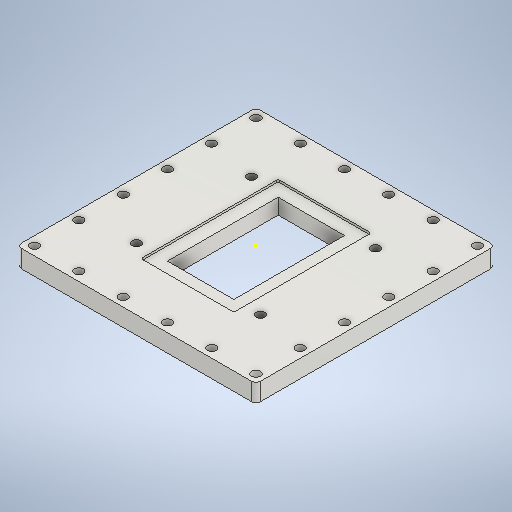
# Autodesk Inventor part: Impact Test Fixturev4 BS EN 6038 assemblyFEA
Saved by Autodesk Inventor 2025 (Build 290162000, 162)
## iProperties
Created: 2024-10-03
Part Number: Impact Test Fixturev4 BS EN 6038 assemblyFEA
Material: Steel, Carbon
Document SubType Name: Modeling
Designer: dr1e22
Density: 7.85 g/cm^3
Appearance: Steel
Author: dr1e22
Autodesk Inventor part; units mm, degrees
ref_plane "YZ Plane" through (0, 0, 0) normal (1, 0, 0) x (0, 1, 0)
ref_plane "XZ Plane" through (0, 0, 0) normal (0, 1, 0) x (-1, 0, 0)
ref_plane "XY Plane" through (0, 0, 0) normal (0, 0, 1) x (1, 0, 0)
sketch "Sketch1" plane through (0, 0, 0) normal (0, 1, 0) x (-1, 0, 0)
  line L0 (130, 135) -> (-130, 135)
  line L1 (-135, 130) -> (-135, -130)
  line L2 (-130, -135) -> (130, -135)
  line L3 (135, -130) -> (135, 130)
  line L4 (135, 135) -> (-135, -135) construction
  line L5 (-135, 135) -> (135, -135) construction
  arc A0 (135, 130) -> (130, 135) centre (130, 130) ccw
  arc A1 (130, -135) -> (135, -130) centre (130, -130) ccw
  arc A2 (-135, -130) -> (-130, -135) centre (-130, -130) ccw
  arc A3 (-130, 135) -> (-135, 130) centre (-130, 130) ccw
  point P0 (0, 0)
  point P1 (0, 0)
  dimension "d0" = 270
  dimension "d1" = 270
  dimension "d2" = 5
  dimension "d3" = 5
  dimension "d4" = 5
  dimension "d5" = 5
  constraints: 12 end point, 8 point on circle, 8 point on line, 8 tangent, 4 centre point, 2 midpoint, 2 parallel, 1 coincident, 1 horizontal, 1 perpendicular
  measures "d0" distance of L4.end L5.end
  measures "d1" distance of L5.end L4.start
  measures "d2" radius of A0
  measures "d3" radius of A1
  measures "d4" radius of A2
  measures "d5" radius of A3
extrude "Extrusion1" add sketch "Sketch1" along normal blind 20
sketch "Sketch2" plane through (0, 20, 0) normal (0, 1, 0) x (1, 0, 0)
  line L0 (-37.5, -62.5) -> (37.5, -62.5)
  line L1 (37.5, -62.5) -> (37.5, 62.5)
  line L2 (37.5, 62.5) -> (-37.5, 62.5)
  line L3 (-37.5, 62.5) -> (-37.5, -62.5)
  line L4 (-37.5, -62.5) -> (37.5, 62.5) construction
  line L5 (37.5, -62.5) -> (-37.5, 62.5) construction
  point P0 (0, 0)
  dimension "d8" = 75
  dimension "d9" = 125
  constraints: 12 end point, 2 midpoint, 2 parallel, 1 horizontal, 1 perpendicular
  measures "d8" distance of L1.end L2.end
  measures "d9" distance of L0.end L1.end
extrude "Extrusion2" cut sketch "Sketch2" against normal blind 65.25
sketch "Sketch3" plane through (0, 20, 0) normal (0, 1, 0) x (1, 0, 0)
  line L0 (-50.5, -77.5) -> (50.5, -77.5)
  line L1 (52.5, -75.5) -> (52.5, 75.5)
  line L2 (50.5, 77.5) -> (-50.5, 77.5)
  line L3 (-52.5, 75.5) -> (-52.5, -75.5)
  line L4 (-52.5, -77.5) -> (52.5, 77.5) construction
  line L5 (52.5, -77.5) -> (-52.5, 77.5) construction
  arc A0 (-50.5, 77.5) -> (-52.5, 75.5) centre (-50.5, 75.5) ccw
  arc A1 (52.5, 75.5) -> (50.5, 77.5) centre (50.5, 75.5) ccw
  arc A2 (50.5, -77.5) -> (52.5, -75.5) centre (50.5, -75.5) ccw
  arc A3 (-52.5, -75.5) -> (-50.5, -77.5) centre (-50.5, -75.5) ccw
  point P0 (0, 0)
  dimension "d12" = 105
  dimension "d13" = 155
  dimension "d14" = 2
  constraints: 12 end point, 8 point on circle, 8 point on line, 8 tangent, 4 centre point, 3 equal radius, 2 midpoint, 2 parallel, 1 horizontal, 1 perpendicular
  measures "d12" distance of L4.end L5.end
  measures "d13" distance of L5.start L4.end
  measures "d14" radius of A0
extrude "Extrusion3" cut sketch "Sketch3" against normal blind 2.5
sketch "Sketch5" plane through (0, 20, 0) normal (0, 1, 0) x (1, 0, 0)
  circle A0 centre (-70, 65) radius 5
  circle A1 centre (70, 65) radius 5
  circle A2 centre (70, -65) radius 5
  circle A3 centre (-70, -65) radius 5
  point P0 (0, 0)
  dimension "d17" = 10
  dimension "d18" = 10
  dimension "d19" = 10
  dimension "d20" = 10
  constraints: 4 centre point
  measures "d17" diameter of A0
  measures "d18" diameter of A1
  measures "d19" diameter of A2
  measures "d20" diameter of A3
hole "Hole1" at (-70, 20, 65) at (-70, 20, -65) at (70, 20, -65) at (70, 20, 65) direction (0, -1, 0) diameter 10 end through all
sketch "Sketch6" plane through (0, 20, 0) normal (0, 1, 0) x (1, 0, 0)
  point P0 (0, 0)
sketch "Sketch7" plane through (0, 20, 0) normal (0, 1, 0) x (1, 0, 0)
  line L0 (-135, 130) -> (-135, -130) projected
  line L1 (130, 135) -> (-130, 135) projected
  line L2 (135, -130) -> (135, 130) projected
  circle A0 centre (70, -65) radius 5 projected
  circle A1 centre (70, 65) radius 5 projected
  circle A2 centre (-70, 65) radius 5 projected
  circle A3 centre (-70, -65) radius 5 projected
  line L3 (52.5, 75.5) -> (52.5, -75.5) projected
  arc A4 (50.5, -77.5) -> (52.5, -75.5) centre (50.5, -75.5) ccw projected
  line L4 (50.5, -77.5) -> (-50.5, -77.5) projected
  arc A5 (-52.5, -75.5) -> (-50.5, -77.5) centre (-50.5, -75.5) ccw projected
  line L5 (-52.5, -75.5) -> (-52.5, 75.5) projected
  arc A6 (-50.5, 77.5) -> (-52.5, 75.5) centre (-50.5, 75.5) ccw projected
  line L6 (-50.5, 77.5) -> (50.5, 77.5) projected
  arc A7 (52.5, 75.5) -> (50.5, 77.5) centre (50.5, 75.5) ccw projected
  arc A8 (130, -135) -> (135, -130) centre (130, -130) ccw projected
  line L7 (135, -130) -> (135, 130) projected
  arc A9 (135, 130) -> (130, 135) centre (130, 130) ccw projected
  line L8 (130, 135) -> (-130, 135) projected
  arc A10 (-130, 135) -> (-135, 130) centre (-130, 130) ccw projected
  line L9 (-135, 130) -> (-135, -130) projected
  arc A11 (-135, -130) -> (-130, -135) centre (-130, -130) ccw projected
  line L10 (-130, -135) -> (130, -135) projected
  circle A12 centre (-125, -125) radius 5
  circle A13 centre (-125, -75) radius 5
  circle A14 centre (-125, -25) radius 5
  circle A15 centre (-125, 25) radius 5
  circle A16 centre (-125, 75) radius 5
  circle A17 centre (-125, 125) radius 5
  circle A18 centre (125, 75) radius 5
  circle A19 centre (125, 25) radius 5
  circle A20 centre (125, -25) radius 5
  circle A21 centre (125, -75) radius 5
  circle A22 centre (125, -125) radius 5
  circle A23 centre (-75, 125) radius 5
  circle A24 centre (75, 125) radius 5
  circle A25 centre (-75, -125) radius 5
  circle A26 centre (75, -125) radius 5
  circle A27 centre (125, 125) radius 5
  circle A28 centre (-25, 125) radius 5
  circle A29 centre (25, 125) radius 5
  circle A30 centre (-25, -125) radius 5
  circle A31 centre (25, -125) radius 5
  point P0 (0, 0)
  point P1 (0, 135)
  point P2 (0, 135)
  dimension "d34" = 10
  dimension "d36" = 10
  dimension "d37" = 10
  dimension "d39" = 10
  dimension "d40" = 10
  dimension "d49" = 50
  dimension "d50" = 50
  dimension "d52" = 50
  dimension "d53" = 50
  dimension "d54" = 10
  dimension "d55" = 10
  dimension "d56" = 10
  dimension "d57" = 10
  dimension "d58" = 10
  dimension "d59" = 50
  dimension "d60" = 10
  dimension "d63" = 10
  dimension "d64" = 10
  dimension "d65" = 10
  dimension "d66" = 10
  dimension "d67" = 10
  dimension "d68" = 10
  dimension "d69" = 10
  dimension "d70" = 10
  dimension "d72" = 10
  dimension "d73" = 10
  dimension "d74" = 10
  dimension "d75" = 50
  dimension "d76" = 10
  dimension "d77" = 50
  dimension "d78" = 10
  dimension "d79" = 50
  dimension "d80" = 10
  dimension "d81" = 10
  dimension "d82" = 10
  dimension "d83" = 50
  dimension "d84" = 50
  dimension "d85" = 10
  dimension "d86" = 50
  dimension "d87" = 75
  dimension "d88" = 50
  dimension "d89" = 10
  dimension "d90" = 75
  dimension "d91" = 10
  dimension "d92" = 50
  dimension "d93" = 50
  dimension "d94" = 10
  dimension "d95" = 10
  dimension "d96" = 10
  dimension "d97" = 10
  dimension "d98" = 10
  dimension "d99" = 50
  dimension "d100" = 50
  dimension "d101" = 50
  dimension "d102" = 10
  dimension "d103" = 10
  dimension "d104" = 10
  dimension "d105" = 10
  dimension "d106" = 50
  dimension "d107" = 50
  dimension "d108" = 50
  constraints: 20 centre point, 2 midpoint
  measures "d34" diameter of A12
  measures "d36" diameter of A13
  measures "d37" diameter of A14
  measures "d39" diameter of A15
  measures "d40" diameter of A16
  measures "d49" distance of A15.centre A16.centre
  measures "d50" distance of A14.centre A15.centre
  measures "d52" distance of A13.centre A14.centre
  measures "d53" distance of A12.centre A13.centre
  measures "d54" distance from line of A12.centre L0
  measures "d55" distance from line of A12.centre L10
  measures "d56" diameter of A17
  measures "d57" distance from line of L1 A17.centre
  measures "d58" distance from line of L9 A17.centre
  measures "d59" distance of A16.centre A17.centre
  measures "d60" diameter of A18
  measures "d63" diameter of A19
  measures "d64" diameter of A20
  measures "d65" diameter of A21
  measures "d66" diameter of A22
  measures "d67" diameter of A23
  measures "d68" diameter of A24
  measures "d69" diameter of A25
  measures "d70" diameter of A26
  measures "d72" diameter of A27
  measures "d73" distance from line of L2 A27.centre
  measures "d74" distance from line of L1 A27.centre
  measures "d75" distance of A27.centre A18.centre
  measures "d76" distance from line of L2 A19.centre
  measures "d77" distance of A18.centre A19.centre
  measures "d78" distance from line of L2 A20.centre
  measures "d79" distance of A20.centre A19.centre
  measures "d80" distance from line of L7 A21.centre
  measures "d81" distance from line of L2 A22.centre
  measures "d82" distance from line of L10 A22.centre
  measures "d83" distance of A20.centre A21.centre
  measures "d84" distance of A21.centre A22.centre
  measures "d85" distance from line of L1 A23.centre
  measures "d86" distance of A17.centre A23.centre
  measures "d87" horizontal distance of point (0, 135) A23.centre
  measures "d88" distance of A27.centre A24.centre
  measures "d89" distance from line of L1 A24.centre
  measures "d90" horizontal distance of point (0, 135) A24.centre
  measures "d91" distance from line of L10 A25.centre
  measures "d92" distance of A12.centre A25.centre
  measures "d93" distance of A22.centre A26.centre
  measures "d94" distance from line of L10 A26.centre
  measures "d95" diameter of A28
  measures "d96" diameter of A29
  measures "d97" diameter of A30
  measures "d98" diameter of A31
  measures "d99" distance of A28.centre A23.centre
  measures "d100" distance of A29.centre A28.centre
  measures "d101" distance of A24.centre A29.centre
  measures "d102" distance from line of L1 A28.centre
  measures "d103" distance from line of L1 A29.centre
  measures "d104" distance from line of L10 A30.centre
  measures "d105" distance from line of L10 A31.centre
  measures "d106" distance of A25.centre A30.centre
  measures "d107" distance of A30.centre A31.centre
  measures "d108" distance of A31.centre A26.centre
hole "Hole2" at (-125, 20, -125) at (-75, 20, -125) at (-25, 20, -125) at (25, 20, -125) at (75, 20, -125) at (125, 20, -125) at (125, 20, -75) at (125, 20, -25) at (125, 20, 25) at (125, 20, 75) at (125, 20, 125) at (75, 20, 125) at (25, 20, 125) at (-25, 20, 125) at (-75, 20, 125) at (-125, 20, 125) at (-125, 20, -75) at (-125, 20, -25) at (-125, 20, 25) at (-125, 20, 75) direction (0, -1, 0) diameter 10 end through all
sketch "Sketch8" plane through (0, 20, 0) normal (0, 1, 0) x (1, 0, 0)
  point P0 (0, 0)
thread "Thread1" size "M10x1.5" class "6H" standard "ANSI Metric M Profile" full length
thread "Thread2" size "M10x1.5" class "6H" standard "ANSI Metric M Profile" full length
thread "Thread3" size "M10x1.5" class "6H" standard "ANSI Metric M Profile" full length
thread "Thread4" size "M10x1.5" class "6H" standard "ANSI Metric M Profile" full length
